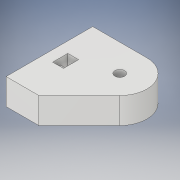
# Autodesk Inventor part: Hopper GUI Corner holder
Saved by Autodesk Inventor 2018 (Build 220112000, 112)
## iProperties
Created: 2013-10-29
Part Number: Hopper GUI Corner holder
Material: Nylon 6/6
Document SubType Name: Modeling
Designer: Gabriel Smolnycki
Mass: 15.4831 g
Surface Area: 46.0858 cm^2
Volume: 13.7019 cm^3
Density: 1.13 g/cm^3
Appearance: Smooth - White
Sending System: SolidWorks 2017
Last Author: Gabriel Smolnycki
Last Saved: 2017-09-14
Author: Gabriel Smolnycki
Autodesk Inventor part; units mm, degrees
ref_plane "YZ Plane" through (0, 0, 0) normal (1, 0, 0) x (0, 1, 0)
ref_plane "XZ Plane" through (0, 0, 0) normal (0, 1, 0) x (-1, 0, 0)
ref_plane "XY Plane" through (0, 0, 0) normal (0, 0, 1) x (1, 0, 0)
sketch "Sketch1" plane through (0, 0, 0) normal (0, 1, 0) x (-1, 0, 0)
  line L0 (9.8223, 27.5) -> (-8.8388, 8.8388)
  line L1 (25, 27.5) -> (9.8223, 27.5)
  line L2 (25, -12.5) -> (25, 27.5)
  line L3 (0, -12.5) -> (25, -12.5)
  arc A0 (-8.8388, 8.8388) -> (0, -12.5) centre (0, 0) ccw
  constraints: 8 end point, 2 horizontal, 2 point on circle, 1 centre point, 1 vertical
extrude "Extrusion4" add sketch "Sketch1" along normal blind 12
sketch "Sketch2" plane through (0, 12, 0) normal (0, 1, 0) x (1, 0, 0)
  point P0 (0, 0)
hole "Hole1" at (0, 12, 0) direction (0, -1, 0) diameter 4.5 depth 12
sketch "Sketch3" plane through (0, 0, 0) normal (0, 1, 0) x (-1, 0, 0)
  line L0 (15, 4) -> (15, 11)
  line L1 (20, 4) -> (15, 4)
  line L2 (15, 11) -> (20, 11)
  line L3 (20, 11) -> (20, 4)
  constraints: 8 end point, 2 horizontal, 2 vertical
extrude "Extrusion3" cut sketch "Sketch3" along normal blind 12
sketch "Sketch4" plane through (-15, 0, 11) normal (-1, 0, 0) x (0, 0, 1)
  line L0 (-3.5, 9.182) -> (-1.909, 7.591)
  arc A0 (-5.091, 7.591) -> (-1.909, 7.591) centre (-3.5, 6) ccw
  line L1 (-5.091, 7.591) -> (-3.5, 9.182)
  constraints: 4 end point, 2 perpendicular, 2 point on circle, 1 centre point
extrude "Extrusion2" cut sketch "Sketch4" against normal blind 10 draft 0
sketch "Sketch5" plane through (-20, 0, 4) normal (1, 0, 0) x (0, 0, -1)
  line L0 (-3.5, 9.182) -> (-1.909, 7.591)
  arc A0 (-5.091, 7.591) -> (-1.909, 7.591) centre (-3.5, 6) ccw
  line L1 (-5.091, 7.591) -> (-3.5, 9.182)
  constraints: 4 end point, 2 perpendicular, 2 point on circle, 1 centre point
extrude "Extrusion1" cut sketch "Sketch5" against normal blind 5
body "Solid3"
